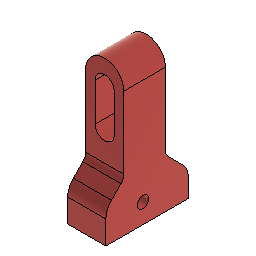
UCF_SlottedTower (Autodesk Fusion 360 archive; units mm, degrees)
design "Tower"
Autodesk Fusion 360 part; units mm, degrees
note: some values were not read from the file. Chosen so that the rebuilt part matches the saved one: which bodies a step acts on; which face or edge a step refers to. Set by a fixed rule: the direction of a hole; which sketch regions a step uses.
sketch "Right" plane through (0, 0, 0) normal (1, 0, 0) x (0, 1, 0) in component "Tower"
  line L0 (0, 0) -> (0, 11.6117)
  line L1 (27.432, 9.9611) -> (27.432, 0)
  arc A0 (27.432, 9.9611) -> (25.5721, 14.4512) centre (21.082, 9.9611) ccw
  arc A1 (1.8541, 16.096) -> (0, 11.6117) centre (6.35, 11.6117) ccw
  arc A2 (5.0391, 19.281) -> (5.969, 21.526) centre (2.794, 21.526) ccw
  line L2 (5.0391, 19.281) -> (1.8541, 16.096)
  line L3 (20.7419, 19.2814) -> (25.5721, 14.4512)
  arc A3 (19.812, 21.5265) -> (20.7419, 19.2814) centre (22.987, 21.5265) ccw
  line L4 (19.812, 51.8592) -> (19.812, 21.5265)
  line L5 (19.812, 51.8592) -> (5.969, 51.8592)
  line L6 (5.969, 21.526) -> (5.969, 51.8592)
  line L7 (0, 0) -> (27.432, 0)
  circle A4 centre (12.3596, 10.3275) radius 1.8986
  line L8 (3.937, 0) -> (3.937, 12.7) construction
  line L9 (22.987, 0) -> (22.987, 12.7) construction
  circle A5 centre (12.3596, 10.3275) radius 12.7 construction
  dimension "d1" = 27.432
  dimension "d4" = 10.3275
  dimension "d5" = 6.35
  dimension "d6" = 6.8309
  dimension "d7" = 3.175
  dimension "d8" = 3.175
  dimension "d9" = 6.35
  dimension "d11" = 30.3327
  dimension "d13" = 13.843
  dimension "d14" = 9.9611
  dimension "d16" = 45
  dimension "d17" = 45
  dimension "d19" = 3.937
  dimension "d20" = 19.05
  dimension "d21" = 4.445
  dimension "d22" = 3.7973
  dimension "d23" = 12.3596
  dimension "d24" = 25.5721
  dimension "d25" = 14.4512
  dimension "d26" = 21.5265
  dimension "d28" = 12.7
  dimension "d29" = 12.7
  dimension "d46" = 16.096
  dimension "d47" = 1.8541
  dimension "d48" = 25.4
  constraint tangent A2 L6
  constraint perpendicular L1 L7
  constraint vertical L6
  constraint horizontal L5
  constraint vertical L4
  constraint horizontal L7
  constraint vertical L0
  constraint coincident L0.start L7.start
  constraint coincident L7 L8.start
  constraint perpendicular L7 L8
  constraint coincident L7 L9.start
  constraint perpendicular L7 L9
  constraint tangent A3 L4
  constraint tangent L0 A1
  constraint tangent A2 L2
  constraint concentric A4 A5
  measures "d1" distance of L0.start L1.end
  measures "d4" vertical distance of L0.start A4.centre
  measures "d5" radius of A0
  measures "d6" distance of A0.end L3.start
  measures "d7" radius of A3
  measures "d8" radius of A2
  measures "d9" radius of A1
  measures "d11" distance of A3.start L4.start
  measures "d13" distance of L4.start L5.end
  measures "d14" distance of L1.start L1.end
  measures "d16" angle of L3 L7
  measures "d17" angle of L2 L7
  measures "d19" distance of L0 L8
  measures "d20" distance of L8 L9
  measures "d21" distance of L1 L9
  measures "d22" diameter of A4
  measures "d23" horizontal distance of L0.start A4.centre
  measures "d24" horizontal distance of L0.start A0.end
  measures "d25" vertical distance of L0.start A0.end
  measures "d26" vertical distance of L0.start A3.start
  measures "d28" distance of L8.start L8.end
  measures "d29" distance of L9.start L9.end
  measures "d46" vertical distance of L0.start A1.start
  measures "d47" horizontal distance of L0.start A1.start
  measures "d48" diameter of A5
extrude "Extrude1" add sketch "Right" along normal mid plane 12.7 in component "Tower"
sketch "Front" plane through (0, 0, 0) normal (0, 1, 0) x (1, 0, 0) in component "Tower"
  line L0 (3.175, -43.9217) -> (3.175, -31.2217)
  arc A0 (3.175, -31.2217) -> (-3.175, -31.2217) centre (0, -31.2217) ccw
  line L1 (-3.175, -31.2217) -> (-3.175, -43.9217)
  arc A1 (-3.175, -43.9217) -> (3.175, -43.9217) centre (0, -43.9217) ccw
  line L2 (0, -43.9217) -> (0, -31.2217) construction
  dimension "d32" = 6.35
  dimension "d33" = 31.2217
  dimension "d34" = 12.7
  dimension "d35" = 3.175
  constraint tangent L0 A0
  constraint tangent A0 L1
  constraint parallel L0 L1
  constraint tangent L1 A1
  constraint tangent L0 A1
  constraint vertical L2
  measures "d32" diameter of A0
  measures "d33" vertical distance of A0.centre origin
  measures "d34" distance of A1.centre A0.centre
  measures "d35" horizontal distance of origin A0.end
extrude "Extrude2" cut sketch "Front" along normal up to surface (19.812 mm away) in component "Tower"
sketch "Bottom" plane through (0, 0, 0) normal (0, 0, 1) x (1, 0, 0) in component "Tower"
  circle A0 centre (0, 3.937) radius 1.8986
  circle A1 centre (0, 22.987) radius 1.8986
  dimension "d38" = 19.05
  dimension "d39" = 3.7973
  dimension "d40" = 3.7973
  dimension "d41" = 3.937
  constraint vertical A0.centre origin
  constraint vertical A0.centre A1.centre
  measures "d38" distance of A0.centre A1.centre
  measures "d39" diameter of A1
  measures "d40" diameter of A0
  measures "d41" distance of origin A0.centre
hole "Hole1" at (0, 22.987, 0) at (0, 3.937, 0) direction (0, 0, 1) diameter 3.7973 depth 14.224 tip angle 118 in component "Tower"
fillet "Fillet1" radius 6.35 2 edges at (-6.35, 12.8905, 51.8592) (6.35, 12.8905, 51.8592) in component "Tower"
move_face "OffsetFaces1" offset -3.81 1 faces at (-4.7814, 16.4899, 0) in component "Tower"
component "Tower" placed x (1, 0, 0) y (0, 1, 0) z (0, 0, 1) at (0, 0, 0)
equation "d39 = d40"

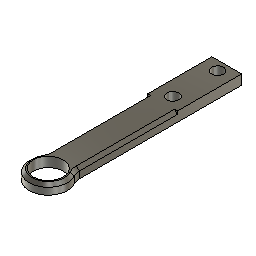
design "UCF_CutterMount_0.75"
Autodesk Fusion 360 part; units mm, degrees
sketch "Sketch1" plane through (0, 0, 0) normal (0, 0, 1) x (1, 0, 0) in component "CutterMount"
  circle A0 centre (0, 0) radius 6.35
  line L0 (-6.35, 6.9514) -> (-6.35, 76.2)
  line L1 (0, 0) -> (0, 76.2) construction
  line L2 (6.35, 6.9514) -> (6.35, 76.2)
  line L3 (-6.35, 76.2) -> (6.35, 76.2)
  arc A1 (-7.1298, 3.9026) -> (7.1298, 3.9026) centre (0, 0) ccw
  circle A2 centre (0, 72.263) radius 2.54
  circle A3 centre (0, 53.213) radius 2.54
  line L4 (-6.35, 48.768) -> (6.35, 48.768)
  arc A4 (6.35, 6.9514) -> (7.1298, 3.9026) centre (12.7, 6.9514) ccw
  arc A5 (-7.1298, 3.9026) -> (-6.35, 6.9514) centre (-12.7, 6.9514) ccw
  dimension "d13_1" = 12.7
  dimension "d16_1" = 6.35
  dimension "d17_1" = 76.2
  dimension "d18_1" = 8.128
  dimension "d19_1" = 5.08
  dimension "d20_1" = 5.08
  dimension "d21_1" = 19.05
  dimension "d198_1" = 3.937
  dimension "d1" = 27.432
  dimension "d2" = 6.35
  constraint coincident A0.centre L1.start
  constraint vertical L0
  constraint parallel L0 L1
  constraint symmetric L0.end L1 L2.end
  constraint coincident L1.end L3
  constraint concentric A0 A1
  constraint coincident L1 A2.centre
  constraint coincident L1 A3.centre
  constraint coincident L0 L4.start
  constraint coincident L2 L4.end
  constraint tangent A1 A4
  constraint tangent L2 A4
  constraint tangent L0 A5
  constraint tangent A1 A5
  constraint equal A4 A5
  measures "d13_1" diameter of A0
  measures "d16_1" distance of A0.centre L0
  measures "d17_1" distance of A0.centre L1.end
  measures "d18_1" radius of A1
  measures "d19_1" diameter of A2
  measures "d20_1" diameter of A3
  measures "d21_1" distance of A2.centre A3.centre
  measures "d198_1" distance of L3 A2.centre
  measures "d2" radius of A4
extrude "Extrude1" add sketch "Sketch1" against normal blind 4.1783 makes body 1 in component "CutterMount"
split "Split2" by curves path "Sketch1" along L4 bodies 1 makes body 2 at (-0.1582, 34.6227, 0) in component "CutterMount"
chamfer "Chamfer3" distance 1.27 angle 45 5 edges at (6.35, 27.8597, 0) (6.548, 5.3779, 0) (0, -8.128, 0) (-6.548, 5.3779, 0) (-6.35, 27.8597, 0) on bodies 2 in component "CutterMount"
combine "Combine2" operation add target body 2 tool bodies 1 in component "CutterMount"
component "CutterMount" placed x (1, 0, 0) y (0, 1, 0) z (0, 0, 1) at (0, 0, 0)
component "CutterMount" placed x (1, 0, 0) y (0, 1, 0) z (0, 0, 1) at (0, 0, 0)

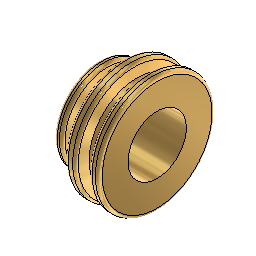
design "DoublePulley"
description: Pulley
Autodesk Fusion 360 part; units mm, degrees
sketch "Sketch2" plane through (0, 0, 0) normal (0, 0, 1) x (1, 0, 0)
  line L0 (-4.9843, -7.493) -> (-5.7409, -9.8217)
  line L1 (-4.9843, -7.493) -> (-3.6995, -7.493)
  line L2 (-3.6995, -7.493) -> (-2.0076, -12.7)
  line L3 (0.7769, -10.414) -> (0.0341, -12.7)
  line L4 (0.7769, -10.414) -> (2.4231, -10.414)
  line L5 (2.4231, -10.414) -> (3.1659, -12.7)
  circle A0 centre (1.6, -12.2784) radius 1.359 construction
  line L6 (3.1659, -12.7) -> (5.1858, -12.7)
  line L7 (-2.0076, -12.7) -> (0.0341, -12.7)
  circle A1 centre (-4.3419, -8.7519) radius 1 construction
  line L8 (-7.5142, -9.8217) -> (-7.5142, -6.35)
  line L9 (-7.5142, 0) -> (5, 0)
  line L10 (-7.5142, -6.35) -> (5.1858, -6.35)
  line L11 (5.1858, -12.7) -> (5.1858, -6.35)
  line L12 (-5.7409, -9.8217) -> (-7.5142, -9.8217)
  dimension "d142_1_1_1" = 12.7
  dimension "d145_1_1_1" = 108
  dimension "d146_1_1_1" = 108
  dimension "d147_1_1_1" = 1.6
  dimension "d150_1_1_1" = 10.414
  dimension "d152_1_1_1" = 12.2784
  dimension "d158_1_1_1" = 12.7
  dimension "d159_1_1_1" = 6.35
  dimension "d161_1_1_1" = 108
  dimension "d162_1_1_1" = 7.493
  dimension "d165_1_1_1" = 108
  dimension "d166_1_1_1" = 2
  dimension "d167_1_1_1" = 7.5142
  dimension "d169_1_1_1" = 9.8217
  dimension "d64_1_1" = 1.6462
  dimension "d65_1_1" = 2.5299
  dimension "d66_1_1" = 2.0418
  constraint perpendicular L10 L11
  constraint tangent L3 A0
  constraint tangent L5 A0
  constraint horizontal L7
  constraint horizontal L6
  constraint parallel L9 L10
  constraint horizontal L1
  constraint vertical L8
  constraint horizontal L12
  constraint tangent L2 A1
  constraint tangent L0 A1
  constraint collinear L6 L7
  constraint horizontal L4
  measures "d142_1_1_1" distance of origin L6
  measures "d145_1_1_1" angle of L3 L4
  measures "d146_1_1_1" angle of L4 L5
  measures "d147_1_1_1" horizontal distance of origin A0.centre
  measures "d150_1_1_1" distance of origin L4
  measures "d152_1_1_1" vertical distance of origin A0.centre
  measures "d158_1_1_1" distance of L10.end L8.end
  measures "d159_1_1_1" distance of origin L10
  measures "d161_1_1_1" angle of L2 L7
  measures "d162_1_1_1" distance of origin L1
  measures "d165_1_1_1" angle of L0 L1
  measures "d166_1_1_1" diameter of A1
  measures "d167_1_1_1" horizontal distance of origin L8.end
  measures "d169_1_1_1" distance of origin L12
  measures "d64_1_1" distance of L3.start L4.end
  measures "d65_1_1" distance of L0.start L8
  measures "d66_1_1" distance of L3.end L2.end
revolve "Revolve2" add sketch "Sketch2" angle 360 about axis through (-7.5142, 0, 0) along (1, 0, 0)
fillet "Fillet1" radius 0.75 6 edges at (-7.5142, -3.5517, -9.1571) (-5.7409, -3.5517, -9.1571) (-2.0076, -4.5925, -11.8406) (0.0341, -4.5925, -11.8406) (3.1659, -4.5925, -11.8406) (5.1858, -4.5925, -11.8406)
equation "d116_1 = 0.0000 in"
equation "d117_1 = 0.0000 in"
equation "d118_1 = 0.0000 in"
equation "d119_1 = 0.000 deg"
equation "d128_1 = 0.0000 in"
equation "d129_1 = 0.0000 in"
equation "d130_1 = 0.0000 in"
equation "d131_1 = 0.000 deg"

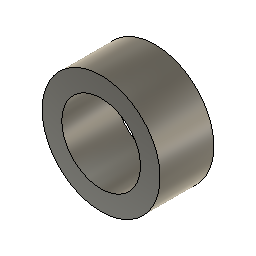
design "Spacer"
description: 1/4" X 3/8" X0.171"
Autodesk Fusion 360 part; units mm, degrees
sketch "Sketch1" plane through (0, 0, 0) normal (0, 1, 0) x (1, 0, 0)
  circle A0 centre (0, 0) radius 3.175
  circle A1 centre (0, 0) radius 4.7625
  dimension "d1" = 6.35
  dimension "d2" = 9.525
  constraint coincident A0.centre A1.centre
  constraint concentric A0 A1
  measures "d1" diameter of A0
  measures "d2" diameter of A1
extrude "Extrude1" add sketch "Sketch1" along normal blind 4.3434
